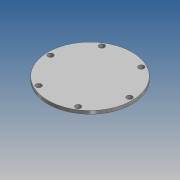
# Autodesk Inventor part: P019
Saved by Autodesk Inventor 2021.4 (Build 254397000, 397)
## iProperties
Created: 2022-05-29
Part Number: P019
Material: Aluminium
Document SubType Name: Modeling
Designer: Rémi Heredero
Density: 2.7 g/cm^3
Appearance: Aluminum - Dark
Author: Rémi Heredero
Title: Chapeau Tete Chambre
Autodesk Inventor part; units mm, degrees
ref_plane "YZ Plane" through (0, 0, 0) normal (1, 0, 0) x (0, 1, 0)
ref_plane "XZ Plane" through (0, 0, 0) normal (0, 1, 0) x (-1, 0, 0)
ref_plane "XY Plane" through (0, 0, 0) normal (0, 0, 1) x (1, 0, 0)
sketch "Sketch2" plane through (0, 0, 0) normal (0, 0, 1) x (1, 0, 0)
  circle A0 centre (0, 0) radius 26.5
  dimension "d0" = 53
  constraints: 1 centre point, 1 coincident
  measures "d0" diameter of A0
extrude "Extrusion1" add sketch "Sketch2" along normal blind 2
sketch "Sketch3" plane through (0, 0, 2) normal (0, 0, 1) x (1, 0, 0)
  circle A0 centre (-12.8301, 20.2827) radius 1.2295 construction
  circle A1 centre (-11.1503, -21.2526) radius 1.2295 construction
  circle A2 centre (23.9804, 0.9699) radius 1.2295 construction
  circle A3 centre (12.8301, -20.2827) radius 1.2295 construction
  circle A4 centre (-23.9804, -0.9699) radius 1.2295 construction
  circle A5 centre (11.1503, 21.2526) radius 1.2295 construction
  circle A6 centre (0, 0) radius 26.5 construction
  circle A7 centre (0, 0) radius 21.5 projected
  point P0 (0, 0)
hole "Hole1" at (23.9804, 0.9699, 2) at (12.8301, -20.2827, 2) at (-11.1503, -21.2526, 2) at (-23.9804, -0.9699, 2) at (-12.8301, 20.2827, 2) at (11.1503, 21.2526, 2) direction (0, 0, -1) diameter 3.4 end through all clearance for "Countersunk Flat Head Screw ISO 2009/7046" size "M3" standard "ISO"
sketch "Sketch4" plane through (0, 0, 0) normal (0, 0, -1) x (-1, 0, 0)
  circle A0 centre (-7.3947, 4.6777) radius 2.5
  circle A1 centre (-7.3947, 4.6777) radius 4.5
  circle A2 centre (-7.3947, 4.6777) radius 6 construction
  point P0 (0, 0)
  dimension "d10" = 5
  dimension "d11" = 2
  constraints: 2 centre point, 1 coincident, 1 concentric
  measures "d10" diameter of A0
  measures "d11" radial gap between concentric circles of A1 A0
extrude "Extrusion2" add sketch "Sketch4" along normal blind 13
chamfer "Chamfer1" distance 1 angle 45 1 edges at (9.8947, 4.6777, -13)
body "Solid1"
